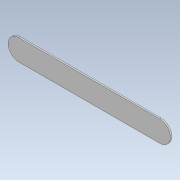
# Autodesk Inventor part: 大臂01
Saved by Autodesk Inventor 2022.5 (Build 265521000, 521)
## iProperties
Created: 2024-11-12
Part Number: 大臂01
Material: 常规
Document SubType Name: Modeling
Designer: Gagouking
Density: 1 g/cm^3
Appearance: 默认
Author: Gagouking
Autodesk Inventor part; units mm, degrees
ref_plane "YZ Plane" through (0, 0, 0) normal (1, 0, 0) x (0, 1, 0)
ref_plane "XZ Plane" through (0, 0, 0) normal (0, 1, 0) x (-1, 0, 0)
ref_plane "XY Plane" through (0, 0, 0) normal (0, 0, 1) x (1, 0, 0)
sketch "草图1" plane through (0, 0, 0) normal (0, 0, 1) x (1, 0, 0)
  line L0 (0, 0) -> (100, 0) construction
  line L1 (0, -7.5) -> (100, -7.5)
  line L2 (100, 7.5) -> (0, 7.5)
  arc A0 (0, 7.5) -> (0, -7.5) centre (0, 0) ccw
  arc A1 (100, -7.5) -> (100, 7.5) centre (100, 0) ccw
  point P0 (50, 0)
  dimension "d1" = 100
  dimension "d4" = 7.5
  constraints: 8 end point, 4 point on circle, 4 tangent, 2 centre point, 1 horizontal, 1 midpoint, 1 parallel
  measures "d1" distance of L0.start L0.end
  measures "d4" radius of A0
extrude "拉伸1" add sketch "草图1" along normal blind 1
